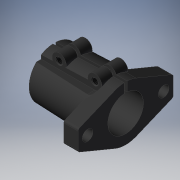
# Autodesk Inventor part: SHFTL30_b
Saved by Autodesk Inventor 2019 (Build 230136000, 136)
## iProperties
Created: 2022-11-15
Part Number: SHFTL30_b
Material: Generic
Catalog Web Link: www.cadenas.de
Description: SHFTL, SHFML, SHFSSL, SHFL_b-Shaft Supports - Flanged Type (Precision Casting) - Long Guide Type
Vendor: MISUMI
Document SubType Name: Modeling
Designer: psAdmin
Manufacturer: MISUMI
Mass: 60.6646 g
Surface Area: 206.307 cm^2
Volume: 60.6646 cm^3
Density: 1 g/cm^3
Appearance: PSOLRGB-175-175-175
Category: PARTsolutions
Company: MISUMI
Title: SHFTL30
Author: Cadenas PARTsolutions
Comments: Shaft Supports - Flanged Type (Precision Casting) - Long Guide Type
PSOL_IDENT_0: {$CADENAS_DATA/23d-libs/misumi/metric/02_shaft_supports/shftl/shftl_b.prj},185 {VTYP=3D},{NB=SHFTL30
PSOL_IDENT_1: _b},{LINA=SHFTL30},{NN=SHFTL, SHFML, SHFSSL, SHFL_b},{DATE=30.03.2018 01:12:37},{GEOMDATE=20.05.2016
PSOL_IDENT_2: 05:12:00},{VERSION=},{LINEID=190},{WBVAR=MAT,ST},{WBNUMERIC=}  {NB=SHFTL30_b},{LINA=SHFTL30},{KT=DU
PSOL_IDENT_3: MMY},{PN=SHFTL30},{TYPE=SHFTL},{MAT=1045},{ST=Black Oxide},{AC=Hexagon Socket Head Cap Screws 2 Pcs.
PSOL_IDENT_4: },{D=30},{L=80},{T=60},{TT=12},{H=50.0},{A=46},{L1=64},{DD=9.0},{DD1=12},{D1=35},{TT1=2.0},{B=22},{C=
PSOL_IDENT_5: 2.5},{BB1=0},{BB2=0},{BB3=0},{HH=21.0},{G=15.0},{F=30},{M=M6},{THMD=6},{THDMIN=0.000},{ST0='Black Ox
PSOL_IDENT_6: ide','Black Oxide','Electroless Nickel Plating','Electroless Nickel Plating'},{MASS=450},{MAT1='1045'
PSOL_IDENT_7: ,'1045 Carbon Steel','514','Aluminum Casting Alloy 514.0','304','304 Stainless Steel'},{DM=6},{HM=20
PSOL_IDENT_8: .000},{MASSS=450},{MASSA=156}
NB: SHFTL30_b
NN: SHFTL, SHFML, SHFSSL, SHFL_b
NT: Shaft Supports - Flanged Type (Precision Casting) - Long Guide Type
NBSYN: $PN._b
LINA: SHFTL30
CATALOG: Misumi
PN: SHFTL30
MAT: 1045 Carbon Steel
ST: Black Oxide
D: 30
L: 80
T: 60
TT: 12
H: 50
A: 46
L1: 64
DD: 9
DD1: 12
D1: 35
TT1: 2
B: 22
C: 2.5
HH: 21
G: 15
F: 30
M: M6
MASS: 450
SUPPLIER: MISUMI
ARTICLENO: SHFTL30_b
BOMINFO: SHFTL30
CREATOR: CADENAS GmbH
Autodesk Inventor part; units mm, degrees
sketch "Sketch_1" plane through (0, 0, 0) normal (1, 0, 0) x (0, 1, 0)
  arc A0 (-6.9901, 40) -> (-8.8379, 38.7654) centre (-6.9901, 38) ccw
  line L0 (-8.8379, 38.7654) -> (-21.2492, 8.8017)
  arc A1 (-21.2492, 8.8017) -> (-21.2492, -8.8017) centre (0, 0) ccw
  line L1 (-21.2492, -8.8017) -> (-8.8379, -38.7654)
  arc A2 (-8.8379, -38.7654) -> (-6.9901, -40) centre (-6.9901, -38) ccw
  line L2 (-6.9901, -40) -> (6.9901, -40)
  arc A3 (6.9901, -40) -> (8.8379, -38.7654) centre (6.9901, -38) ccw
  line L3 (8.8379, -38.7654) -> (21.2492, -8.8017)
  arc A4 (21.2492, -8.8017) -> (21.2492, 8.8017) centre (0, 0) ccw
  line L4 (21.2492, 8.8017) -> (8.8379, 38.7654)
  arc A5 (8.8379, 38.7654) -> (6.9901, 40) centre (6.9901, 38) ccw
  line L5 (6.9901, 40) -> (-6.9901, 40)
  constraints: 12 end point, 12 point on circle, 6 centre point
extrude "Extrusion1" add sketch "Sketch_1" against normal blind 12
sketch "_____1" plane through (-12, 0, 0) normal (1, 0, 0) x (0, 0, -1)
  circle A0 centre (0, 0) radius 22.975
  constraints: 1 centre point
extrude "Extrusion2" add sketch "_____1" against normal blind 48 draft -2
sketch "Sketch_3" plane through (0, 0, -11) normal (0, 0, 1) x (1, 0, 0)
  circle A0 centre (-15, 21) radius 6
  constraints: 1 centre point
extrude "Extrusion3" add sketch "Sketch_3" along normal blind 23
sketch "Sketch_13" plane through (0, 0, 0) normal (0, 0, 1) x (1, 0, 0)
  circle A0 centre (-45, 21) radius 6
  constraints: 1 centre point
extrude "Extrusion4" add sketch "Sketch_13" along normal mid plane 22
sketch "Sketch_4" plane through (0, 0, 11) normal (0, 0, 1) x (1, 0, 0)
  line L0 (-60, 15) -> (-15, 15)
  arc A0 (-15, 15) -> (-21, 21) centre (-15, 21) ccw
  line L1 (-21, 21) -> (-60, 21)
  line L2 (-60, 21) -> (-60, 15)
  constraints: 6 end point, 2 point on circle, 1 centre point
extrude "Extrusion5" cut sketch "Sketch_4" along normal blind 11
sketch "Sketch_5" plane through (0, 0, 0) normal (1, 0, 0) x (0, 1, 0)
  line L0 (50, 1.25) -> (0, 1.25)
  line L1 (0, 1.25) -> (0, -1.25)
  line L2 (0, -1.25) -> (50, -1.25)
  line L3 (50, -1.25) -> (50, 1.25)
  constraints: 8 end point
extrude "Extrusion6" cut sketch "Sketch_5" against normal blind 60
sketch "Sketch_6" plane through (0, 0, 0) normal (0, 0, 1) x (1, 0, 0)
  line L0 (0, 0) -> (-60, 0)
  line L1 (-60, 0) -> (-60, 17.5)
  line L2 (-60, 17.5) -> (-58, 17.5)
  line L3 (-58, 17.5) -> (-58, 15)
  line L4 (-58, 15) -> (0, 15)
  line L5 (0, 15) -> (0, 0)
  line L6 (0, 0) -> (-60, 0)
  constraints: 14 end point
revolve "Revolution1" cut sketch "Sketch_6" angle 360 about axis through (0, 0, 0) along (1, 0, 0)
sketch "Sketch_7" plane through (-15, 0, 0) normal (1, 0, 0) x (0, 0, -1)
  line L0 (16.5, 21) -> (1.25, 21)
  line L1 (1.25, 21) -> (1.25, 24)
  line L2 (1.25, 24) -> (1.7915, 23.4585)
  line L3 (1.7915, 23.4585) -> (10.4585, 23.4585)
  line L4 (10.4585, 23.4585) -> (11, 24)
  line L5 (11, 24) -> (16.5, 24)
  line L6 (16.5, 24) -> (16.5, 21)
  line L7 (16.5, 21) -> (1.25, 21)
  constraints: 16 end point
revolve "Revolution2" cut sketch "Sketch_7" angle 360 about axis through (-15, 21, -16.5) along (0, 0, -1)
thread "Thread1" size "M6x1" class "6H" standard "ISO Metric profile" full length
sketch "Sketch_8" plane through (-15, 0, 0) normal (1, 0, 0) x (0, 0, -1)
  line L0 (-1.25, 21) -> (-11, 21)
  line L1 (-11, 21) -> (-11, 24)
  line L2 (-11, 24) -> (-10.4585, 23.4585)
  line L3 (-10.4585, 23.4585) -> (-1.7915, 23.4585)
  line L4 (-1.7915, 23.4585) -> (-1.25, 24)
  line L5 (-1.25, 24) -> (-1.25, 21)
  line L6 (-1.25, 21) -> (-11, 21)
  constraints: 14 end point
revolve "Revolution3" cut sketch "Sketch_8" angle 360 about axis through (-15, 21, 1.25) along (0, 0, -1)
thread "Thread2" size "M6x1" class "6H" standard "ISO Metric profile" full length
sketch "Sketch10" plane through (0, 0, 0) normal (1, 0, 0) x (0, 0, -1)
  point P0 (32, 0)
hole "Hole1" at (0, 0, -32) direction (-1, 0, 0) diameter 9 depth 12
sketch "Sketch11" plane through (0, 0, 0) normal (1, 0, 0) x (0, 0, -1)
  point P0 (-32, 0)
hole "Hole2" at (0, 0, 32) direction (-1, 0, 0) diameter 9 depth 12
sketch "Sketch_14" plane through (-45, 0, 0) normal (1, 0, 0) x (0, 0, -1)
  line L0 (16.5, 21) -> (1.25, 21)
  line L1 (1.25, 21) -> (1.25, 24)
  line L2 (1.25, 24) -> (1.7915, 23.4585)
  line L3 (1.7915, 23.4585) -> (10.4585, 23.4585)
  line L4 (10.4585, 23.4585) -> (11.1, 24.1)
  line L5 (11.1, 24.1) -> (16.5, 24.1)
  line L6 (16.5, 24.1) -> (16.5, 21)
  line L7 (16.5, 21) -> (1.25, 21)
  constraints: 16 end point
revolve "Revolution4" cut sketch "Sketch_14" angle 360 about axis through (-45, 21, -16.5) along (0, 0, -1)
thread "Thread3" size "M6x1" class "6H" standard "ISO Metric profile" full length
sketch "Sketch_15" plane through (-45, 0, 0) normal (1, 0, 0) x (0, 0, -1)
  line L0 (-1.25, 21) -> (-11, 21)
  line L1 (-11, 21) -> (-11, 24)
  line L2 (-11, 24) -> (-10.4585, 23.4585)
  line L3 (-10.4585, 23.4585) -> (-1.7915, 23.4585)
  line L4 (-1.7915, 23.4585) -> (-1.25, 24)
  line L5 (-1.25, 24) -> (-1.25, 21)
  line L6 (-1.25, 21) -> (-11, 21)
  constraints: 14 end point
revolve "Revolution5" cut sketch "Sketch_15" angle 360 about axis through (-45, 21, 1.25) along (0, 0, -1)
thread "Thread4" size "M6x1" class "6H" standard "ISO Metric profile" full length
ref_plane "body_screw_XY" through (-15, 21, 11) normal (0, 0, 1) x (1, 0, 0)
ref_plane "body_screw_YZ" through (-15, 21, 11) normal (1, 0, 0) x (0, 1, 0)
ref_plane "body_screw_ZX" through (-15, 21, 11) normal (0, 1, 0) x (0, 0, 1)
ref_plane "body_to_screw2_XY" through (-45, 21, 11) normal (0, 0, 1) x (1, 0, 0)
ref_plane "body_to_screw2_YZ" through (-45, 21, 11) normal (1, 0, 0) x (0, 1, 0)
ref_plane "body_to_screw2_ZX" through (-45, 21, 11) normal (0, 1, 0) x (0, 0, 1)
body "Solid1"
